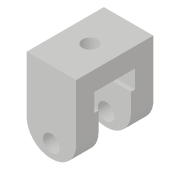
# Autodesk Inventor part: omni wheel wheel holder proto
Saved by Autodesk Inventor 2018 (Build 220112000, 112)
## iProperties
Created: 2019-01-03
Part Number: omni wheel wheel holder proto
Material: Generic
Document SubType Name: Modeling
Designer: ball
Density: 1 g/cm^3
Appearance: Default
Author: ball
Autodesk Inventor part; units mm, degrees
ref_plane "YZ Plane" through (0, 0, 0) normal (1, 0, 0) x (0, 1, 0)
ref_plane "XZ Plane" through (0, 0, 0) normal (0, 1, 0) x (-1, 0, 0)
ref_plane "XY Plane" through (0, 0, 0) normal (0, 0, 1) x (1, 0, 0)
sketch "Sketch1" plane through (0, 0, 0) normal (0, 0, 1) x (1, 0, 0)
  line L0 (6.5024, 2.8448) -> (6.5024, 17.6276)
  line L1 (6.5024, 17.6276) -> (-6.5024, 17.6276)
  line L2 (-6.5024, 2.8448) -> (-6.5024, 17.6276)
  circle A0 centre (0, 0) radius 3.5052 construction
  line L3 (0.1524, -3.5052) -> (-0.1524, -3.5052)
  arc A1 (-6.5024, 2.8448) -> (-0.1524, -3.5052) centre (-0.1524, 2.8448) ccw
  arc A2 (0.1524, -3.5052) -> (6.5024, 2.8448) centre (0.1524, 2.8448) ccw
  circle A3 centre (0, 0) radius 2.1844
  circle A4 centre (0, 0) radius 6.5024 construction
  dimension "d3" = 13.0048
  dimension "d5" = 7.0104
  dimension "d6" = 6.35
  dimension "d7" = 4.3688
  dimension "d10" = 13.0048
  dimension "d11" = 17.6276
  constraints: 8 end point, 5 centre point, 4 point on circle, 3 coincident, 2 tangent, 1 equal radius
  measures "d3" distance between parallel lines of L0 L2
  measures "d5" diameter of A0
  measures "d6" radius of A1
  measures "d7" diameter of A3
  measures "d10" diameter of A4
  measures "d11" distance from line of L1 point (0, 0)
extrude "Extrusion1" add sketch "Sketch1" along normal blind 20.32
sketch "Sketch2" plane through (6.5024, 2.8448, 0) normal (1, 0, 0) x (0, 0, -1)
  line L0 (-20.32, 0) -> (-20.32, 14.7828) construction
  line L1 (-20.32, 9.7028) -> (0, 9.7028) construction
  line L2 (0, 14.7828) -> (-20.32, 14.7828) construction
  line L3 (-20.32, 4.9276) -> (0, 4.9276) construction
  line L4 (0, 14.7828) -> (0, 0) construction
  line L5 (0, 0) -> (-20.32, 0) construction
  line L6 (0, -0.6604) -> (-20.32, -0.6604) construction
  line L7 (0, -5.0292) -> (-20.32, -5.0292) construction
  line L8 (0, -0.6604) -> (0, -5.0292) construction
  line L9 (0, -6.35) -> (0, 0) construction
  line L10 (-10.16, 14.7828) -> (-10.16, -6.35) construction
  line L11 (0, -6.35) -> (-20.32, -6.35) construction
  line L12 (-5.9055, 4.9276) -> (-5.9055, -6.35)
  line L13 (-5.9055, -6.35) -> (-10.16, -6.35)
  line L14 (-14.4145, 4.9276) -> (-14.4145, -6.35)
  line L15 (-14.4145, -6.35) -> (-10.16, -6.35)
  line L16 (-10.16, 9.7028) -> (-4.826, 9.7028)
  line L17 (-4.826, 9.7028) -> (-4.826, 4.9276)
  line L18 (-10.16, 9.7028) -> (-15.494, 9.7028)
  line L19 (-15.494, 9.7028) -> (-15.494, 4.9276)
  line L20 (-15.494, 4.9276) -> (-14.4145, 4.9276)
  line L21 (-4.826, 4.9276) -> (-5.9055, 4.9276)
  point P0 (0, -2.8448)
  dimension "d12" = 5.08
  dimension "d14" = 7.7724
  dimension "d15" = 4.2545
  dimension "d16" = 4.2545
  constraints: 28 end point, 8 point on line, 4 horizontal, 3 collinear, 3 midpoint, 2 perpendicular
  measures "d12" distance between parallel lines of L2 L1
  measures "d14" distance from line of point (0, -2.845) L3
  measures "d15" distance of L13.end L12.end
  measures "d16" distance of L13.end L14.end
extrude "Extrusion2" cut sketch "Sketch2" against normal through all
sketch "Sketch3" plane through (-6.5024, 17.6276, 0) normal (0, 1, 0) x (1, 0, 0)
  line L0 (6.6548, -14.4145) -> (6.6548, -20.32) construction
  line L1 (0, 0) -> (13.0048, 0) construction
  line L2 (6.5024, 0) -> (6.5024, -20.32) construction
  line L3 (13.0048, -20.32) -> (0, -20.32) construction
  line L4 (13.0048, 0) -> (13.0048, -20.32) construction
  line L5 (13.0048, -10.16) -> (0, -10.16) construction
  line L6 (0, 0) -> (0, -20.32) construction
  circle A0 centre (6.5024, -10.16) radius 1.9685 construction
  point P0 (6.5024, 0)
  dimension "d21" = 6.5024
  dimension "d22" = 10.16
  dimension "d23" = 3.937
  constraints: 5 midpoint, 4 end point, 1 centre point, 1 vertical
  measures "d21" distance between parallel lines of L2 L4
  measures "d22" distance between parallel lines of L5 L3
  measures "d23" diameter of A0
hole "Hole1" at (0, 17.6276, 10.16) direction (0, -1, 0) diameter 3.937 end through all
body "Solid1"
